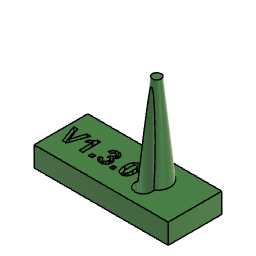
StrawThermocoupleFastener_V1.3.0 (Autodesk Fusion 360 design; units mm, degrees)
Autodesk Fusion 360 part; units mm, degrees
sketch "Sketch1" plane through (0, 0, 0) normal (0, 0, 1) x (1, 0, 0) in component "Component"
  circle A0 centre (0, 0) radius 1.5
  dimension "d1" = 3
  constraint coincident A0.centre origin
  measures "d1" diameter of A0
ref_plane "WorkPlane1" through (0, 0, 10) normal (0, 0, 1) x (1, 0, 0) in component "Component"
sketch "Sketch2" plane through (0, 0, 10) normal (0, 0, 1) x (1, 0, 0) in component "Component"
  circle A0 centre (0, 0) radius 0.5
  dimension "d3" = 1
  constraint coincident A0.centre origin
  measures "d3" diameter of A0
loft "Loft1" add profiles "Sketch1", "Sketch2" section 1 section 2 makes body 1 in component "Component"
sketch "Sketch3" plane through (0, 0, 0) normal (0, 0, -1) x (1, 0, 0) in component "Component"
  circle A0 centre (0, 0) radius 1.5
  line L0 (2.5, -2.5) -> (-2.5, -2.5)
  line L1 (-2.5, 2.5) -> (2.5, 2.5)
  line L2 (0, 0) -> (0.2762, 0)
  line L3 (4.7762, 2.5) -> (4.7762, -2.5)
  line L4 (4.7762, -2.5) -> (-10.2238, -2.5)
  line L5 (-10.2238, -2.5) -> (-10.2238, 2.5)
  line L6 (-10.2238, 2.5) -> (4.7762, 2.5)
  circle A1 centre (0, 1.5) radius 0.75
  dimension "d5" = 15
  dimension "d6" = 1.5
  constraint horizontal L0
  constraint parallel L0 L1
  constraint coincident A0.centre L2.start
  constraint horizontal L2
  constraint perpendicular L3 L4
  constraint parallel L3 L5
  constraint parallel L4 L6
  measures "d5" distance of L3.start L5.end
  measures "d6" diameter of A1
extrude "Extrude2" add sketch "Sketch3" along normal blind 2.75 separate body contours A0 A1 | A0 A1 | L0 L1 L3 L4 L5 L6 picked at (0.0474, -0.7462) picked at (0, 1.2474) makes body 2 in component "Component"
extrude "Extrude3" add sketch "Sketch3" along normal blind 2.75 contours A0 A1 picked at (0.0474, -0.7462) bodies 1 2 in component "Component"
sketch "Sketch4" plane through (0, 0, -2.75) normal (0, 0, -1) x (1, 0, 0) in component "Component"
  line L0 (-10.2238, 2.5) -> (-10.2238, -2.5)
  line L1 (-10.2238, -2.5) -> (4.7762, -2.5)
  line L2 (4.7762, -2.5) -> (4.7762, 2.5)
  line L3 (4.7762, 2.5) -> (-10.2238, 2.5)
  circle A0 centre (0, 1.5) radius 0.9262
  arc A1 (0.7262, 1.3125) -> (-0.7262, 1.3125) centre (0, 1.5) ccw
  arc A2 (0.7262, 1.3125) -> (-0.7262, 1.3125) centre (0, 0) ccw
  constraint concentric A0 A1
extrude "Extrude4" cut sketch "Sketch4" against normal blind 13.3 contours A0 bodies 1 in component "Component"
extrude "Extrude5" add 1 faces at (-5.2238, -2.5, -0.9167) along direction (0, -1, 0) blind 1 on bodies 1 bodies 1 in component "Component"
extrude "Extrude6" cut 1 faces at (-7.1211, -0.7873, -2.75) along direction (0, 0, 1) blind 0.5 on bodies 1 bodies 1 in component "Component"
sketch "Sketch1 (2)" plane through (0, 0, 0) normal (0, 0, 1) x (-1, 0, 0)
  arc A0 (0.881, 1.214) -> (-0.881, 1.214) centre (0, 1.5) ccw
  arc A1 (-0.881, 1.214) -> (0.881, 1.214) centre (0, 0) ccw
  line L0 (10.2238, -2.5) -> (10.2238, 3.5)
  line L1 (10.2238, 3.5) -> (-4.7762, 3.5)
  line L2 (-4.7762, 3.5) -> (-4.7762, -2.5)
  line L3 (-4.7762, -2.5) -> (10.2238, -2.5)
  line L4 (9.025, 1.5079) -> (2.5153, 1.4599) construction
  line L5 (2.5153, 1.4599) -> (2.5298, -0.5079) construction
  line L6 (2.5298, -0.5079) -> (9.0395, -0.4599) construction
  line L7 (9.0395, -0.4599) -> (9.025, 1.5079) construction
  line L8 (10.2238, -2.5) -> (10.2238, 3.5)
  line L9 (10.2238, 3.5) -> (10.2238, 0.5)
  line L10 (10.2238, 0.5) -> (-4.7762, 0.5)
  dimension "d22" = 2
  text T0 "V1.3.0" font "Arial" height 2 bold align centre middle in box 6.5099 x 1.9678 at (9.025, 1.5079) x (-0.999973, -0.007371) y (0.007371, -0.999973) spacing 1 kerned
  constraint coincident L0.start L3.end
  constraint coincident L0.end L1.start
  constraint midpoint L0 L9.end
  constraint midpoint L2 L10.end
  constraint coincident L10
extrude "Extrude8" cut sketch "Sketch1 (2)" against normal blind 0.5 text T0 bodies 1 in component "Component"
component "Component" placed x (1, 0, 0) y (0, 1, 0) z (0, 0, 1) at (0, 0, 0)
